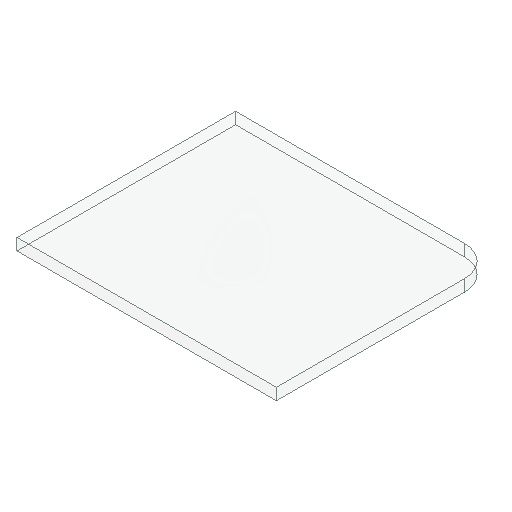
# Autodesk Inventor part: Plexi-glass
Saved by Autodesk Inventor 2025 (Build 290162000, 162)
## iProperties
Created: 2025-01-02
Part Number: Plexi-glass
Material: Glass
Document SubType Name: Modeling
Designer: Jan Mareš
Density: 2.18 g/cm^3
Appearance: Clear
Author: Jan Mareš
Autodesk Inventor part; units mm, degrees
ref_plane "YZ Plane" through (0, 0, 0) normal (1, 0, 0) x (0, 1, 0)
ref_plane "XZ Plane" through (0, 0, 0) normal (0, 1, 0) x (-1, 0, 0)
ref_plane "XY Plane" through (0, 0, 0) normal (0, 0, 1) x (1, 0, 0)
sketch "Sketch1" plane through (0, 0, 0) normal (0, 1, 0) x (-1, 0, 0)
  line L0 (35, 0) -> (-35, 0) construction
  line L1 (0, -28) -> (0, 28) construction
  line L2 (-25, 20) -> (25, 20)
  line L3 (25, 20) -> (25, -20)
  line L4 (25, -20) -> (-25, -20)
  line L5 (-25, -20) -> (-25, 20)
  line L6 (-25, 0) -> (25, 0) construction
  point P0 (0, 0)
  dimension "d0" = 50
  dimension "d1" = 40
  constraints: 10 end point, 3 midpoint, 2 parallel, 1 horizontal, 1 perpendicular
  measures "d0" distance of L2.start L2.end
  measures "d1" distance of L4.end L2.start
extrude "Extrusion1" add sketch "Sketch1" along normal blind 2
sketch "Sketch2" plane through (0, 0, 0) normal (0, -1, 0) x (1, 0, 0)
  line L0 (22.5, 19) -> (22.5, -13.4999) construction
  arc A0 (16.9999, -19) -> (22.5, -13.4999) centre (16.9999, -13.4999) ccw construction
  line L1 (16.9999, -19) -> (-22.5, -19) construction
  line L2 (-22.5, -19) -> (-22.5, 19) construction
  line L3 (-22.5, 19) -> (22.5, 19) construction
  line L4 (-22.25, -18.75) -> (16.9999, -18.75)
  arc A1 (16.9999, -18.75) -> (22.25, -13.4999) centre (16.9999, -13.4999) ccw
  line L5 (22.25, -13.4999) -> (22.25, 18.75)
  line L6 (22.25, 18.75) -> (-22.25, 18.75)
  line L7 (-22.25, 18.75) -> (-22.25, -18.75)
  line L8 (16.9999, -26.75) -> (-30.25, -26.75)
  line L9 (-30.25, -26.75) -> (-30.25, 26.75)
  line L10 (-30.25, 26.75) -> (30.25, 26.75)
  line L11 (30.25, 26.75) -> (30.25, -13.4999)
  arc A2 (16.9999, -26.75) -> (30.25, -13.4999) centre (16.9999, -13.4999) ccw
  point P0 (0, 0)
  dimension "d5" = 0.25
  dimension "d8" = 8
  constraints: 16 end point, 4 point on circle, 2 centre point, 8 other
  measures "d5" distance between parallel lines of L1 L4
  measures "d8" distance between parallel lines of L4 L8
extrude "Extrusion2" cut sketch "Sketch2" against normal up to next
body "Solid1"
